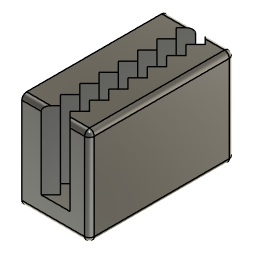
belt lock (Autodesk Fusion 360 design; units mm, degrees)
Autodesk Fusion 360 part; units mm, degrees
sketch "Esquisse1" plane through (0, 0, 0) normal (0, 0, 1) x (1, 0, 0)
  line L0 (2, 0) -> (3.5, 0)
  line L1 (3.5, 0) -> (3.5, 15)
  line L2 (3.5, 15) -> (2, 15)
  line L3 (3.5, 0) -> (5.5, 0)
  line L4 (5.5, 0) -> (5.5, 15)
  line L5 (5.5, 15) -> (3.5, 15)
  line L6 (3.5, 15) -> (3.5, 0)
  line L7 (3.5, 15) -> (2.5, 15)
  line L8 (3.5, 15) -> (3.5, 14)
  line L9 (2.5, 15) -> (3.5, 14)
  line L10 (2.5, 13) -> (3.5, 14)
  line L11 (2.5, 13) -> (3.5, 12)
  line L12 (2.5, 11) -> (3.5, 12)
  line L13 (2.5, 7) -> (3.5, 8)
  line L14 (2.5, 9) -> (3.5, 8)
  line L15 (2.5, 9) -> (3.5, 10)
  line L16 (2.5, 11) -> (3.5, 10)
  line L17 (2.5, 1) -> (3.5, 0)
  line L18 (2.5, 1) -> (3.5, 2)
  line L19 (2.5, 3) -> (3.5, 2)
  line L20 (2.5, 3) -> (3.5, 4)
  line L21 (2.5, 5) -> (3.5, 4)
  line L22 (2.5, 5) -> (3.5, 6)
  line L23 (2.5, 7) -> (3.5, 6)
  line L24 (1.5, 7) -> (0.5, 8)
  line L25 (0.5, 15) -> (1.5, 15)
  line L26 (1.5, 9) -> (0.5, 8)
  line L27 (1.5, 15) -> (0.5, 14)
  line L28 (1.5, 11) -> (0.5, 10)
  line L29 (0.5, 15) -> (0.5, 14)
  line L30 (1.5, 1) -> (0.5, 0)
  line L31 (1.5, 5) -> (0.5, 4)
  line L32 (1.5, 3) -> (0.5, 2)
  line L33 (1.5, 7) -> (0.5, 6)
  line L34 (1.5, 13) -> (0.5, 12)
  line L35 (0.5, 0) -> (-1.5, 0)
  line L36 (1.5, 1) -> (0.5, 2)
  line L37 (1.5, 11) -> (0.5, 12)
  line L38 (1.5, 3) -> (0.5, 4)
  line L39 (1.5, 13) -> (0.5, 14)
  line L40 (1.5, 9) -> (0.5, 10)
  line L41 (1.5, 5) -> (0.5, 6)
  line L42 (0.5, 0) -> (0.5, 15)
  line L43 (-1.5, 15) -> (0.5, 15)
  line L44 (0.5, 15) -> (0.5, 0)
  line L45 (-1.5, 0) -> (-1.5, 15)
  line L46 (0.5, 15) -> (2, 15)
  line L47 (2, 0) -> (0.5, 0)
  dimension "d1" = 3.5
  dimension "d2" = 15
  dimension "d3" = 2
  dimension "d5" = 1
  dimension "d6" = 1
  constraint horizontal L0
  constraint vertical L1
  constraint horizontal L2
  constraint horizontal L3
  constraint vertical L4
  constraint horizontal L5
  constraint vertical L6
  constraint perpendicular L6 L7
  constraint perpendicular L5 L8
  measures "d1" distance of origin L0.end
  measures "d2" distance of L0 L2
  measures "d3" distance of L0.end L3.end
  measures "d5" distance of L1.end L7.end
  measures "d6" distance of L1.end L8.end
extrude "Extrusion1" add sketch "Esquisse1" against normal blind 2
extrude "Extrusion2" add sketch "Esquisse1" along normal blind 8 contours L1 L6 L17 L18 | L1 L3 L4 L5 L6 L8 | L30 L36 L42 L44 | L29 L35 L42 L43 L44 L45 | L1 L6 L19 L20 | L32 L38 L42 L44 | L1 L6 L21 L22 | L31 L41 L42 L44 | L1 L6 L13 L23 | L1 L2 L6 L7 L8 L9 | L25 L27 L29 L42 L44 L46 | L24 L33 L42 L44 | L1 L6 L14 L15 | L1 L6 L10 L11 | L34 L39 L42 L44 | L26 L40 L42 L44 | L1 L6 L12 L16 | L28 L37 L42 L44
fillet "Congé1" radius 0.5 10 edges at (5.5, 15, 3) (5.5, 7.5, -2) (2, 15, -2) (5.5, 0, 3) (2, 0, -2) (5.5, 7.5, 8) (4, 15, 8) (0, 15, 8) (4.5, 0, 8) (-0.5, 0, 8)
equation "d1 = ( 1.75 * 2 ) * 1 mm"
